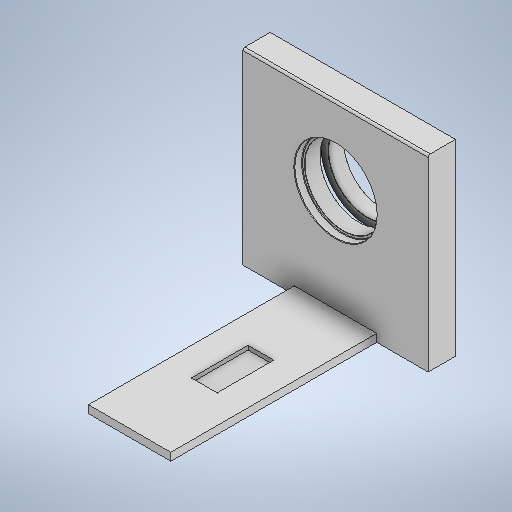
# Autodesk Inventor part: Gantry mssd
Saved by Autodesk Inventor 2025.2 (Build 292293000, 293)
## iProperties
Created: 2025-04-03
Part Number: Gantry mssd
Material: Generic
Document SubType Name: Modeling
Designer: NIKHIL
Density: 1 g/cm^3
Appearance: Default
Author: NIKHIL
Autodesk Inventor part; units mm, degrees
sketch "Sketch1" plane through (0, 0, 0) normal (0, 0, 1) x (1, 0, 0)
  circle A0 centre (0, 0) radius 375
  circle A1 centre (0, 0) radius 450
  dimension "d0" = 750
  dimension "d2" = 900
  constraints: 2 centre point, 2 coincident
  measures "d0" diameter of A0
  measures "d2" diameter of A1
extrude "Extrusion1" add sketch "Sketch1" along normal blind 150
ref_plane "Work Plane1" through (0, 0, -80) normal (0, 0, -1) x (-1, 0, 0)
sketch "Sketch2" plane through (0, 0, -80) normal (0, 0, -1) x (-1, 0, 0)
  circle A0 centre (0, 0) radius 375
  circle A1 centre (0, 0) radius 450
  constraints: 2 centre point, 2 coincident
extrude "Extrusion2" add sketch "Sketch2" along normal blind 150
ref_plane "Work Plane2" through (0, 400, 0) normal (0, 1, 0) x (-1, 0, 0)
sketch "Sketch5" plane through (0, 0, 0) normal (1, 0, 0) x (0, 1, 0)
  line L0 (450, 0) -> (450, 150) projected
  line L1 (450, 70) -> (465, 70)
  line L2 (465, 70) -> (465, 80)
  line L3 (465, 80) -> (450, 80)
  line L4 (450, 80) -> (450, 70)
  line L5 (0, -306) -> (0, 226) projected
  line L6 (450, -80) -> (450, -230) projected
  line L7 (450, -150) -> (465, -150)
  line L8 (465, -150) -> (465, -160)
  line L9 (465, -160) -> (450, -160)
  line L10 (450, -160) -> (450, -150)
  point P0 (0, 0)
  dimension "d11" = 15
  dimension "d12" = 10
  dimension "d14" = 15
  dimension "d15" = 10
  constraints: 16 end point, 4 parallel, 2 horizontal, 2 perpendicular, 2 point on line
  measures "d11" distance of L3.end L2.end
  measures "d12" distance of L2.end L1.end
  measures "d14" distance of L8.end L9.end
  measures "d15" distance of L7.end L8.end
revolve "Revolution1" add sketch "Sketch5" angle 360 about axis through (0, 0, -10) along (0, 0, 1)
ref_plane "Work Plane3" through (0, 0, -40) normal (0, 0, 1) x (1, 0, 0)
ref_plane "Work Plane4" through (0, 0, 150) normal (0, 0, 1) x (1, 0, 0)
sketch "Sketch11" plane through (0, 0, 150) normal (0, 0, 1) x (1, 0, 0)
  circle A0 centre (0, 0) radius 400
  line L0 (-900, 750) -> (900, 750)
  line L1 (900, 750) -> (900, -750)
  line L2 (900, -750) -> (-900, -750)
  line L3 (-900, -750) -> (-900, 750)
  line L4 (-900, 750) -> (900, -750) construction
  line L5 (900, 750) -> (-900, -750) construction
  dimension "d33" = 800
  dimension "d34" = 1800
  dimension "d35" = 1500
  constraints: 12 end point, 2 midpoint, 2 parallel, 1 centre point, 1 coincident, 1 horizontal, 1 perpendicular
  measures "d33" diameter of A0
  measures "d34" distance of L1.end L2.end
  measures "d35" distance of L0.end L1.end
extrude "Extrusion5" add sketch "Sketch11" along normal blind 75
fillet "Fillet1" radius 5 1 edges at (-400, 0, 225)
fillet "Fillet2" radius 5 1 edges at (-400, 0, 150)
fillet "Fillet3" radius 2 1 edges at (-375, 0, 150)
fillet "Fillet4" radius 2 1 edges at (-375, 0, 0)
fillet "Fillet5" radius 2 1 edges at (375, 0, -80)
fillet "Fillet6" radius 2 1 edges at (375, 0, -230)
fillet "Fillet7" radius 2 1 edges at (-450, 0, 0)
fillet "Fillet8" radius 2 2 edges at (450, 0, -80) (450, 0, -230)
fillet "Fillet9" radius 20 1 edges at (0, 750, 225)
sketch "Sketch15" plane through (-900, -750, 150) normal (0, -1, 0) x (1, 0, 0)
  line L0 (1800, 75) -> (1800, 55) projected
  line L1 (0, 0) -> (1800, 0) projected
  line L2 (1800, 75) -> (0, 75)
  line L3 (0, 75) -> (0, 0)
  line L4 (0, 0) -> (1800, 0)
  line L5 (1800, 0) -> (1800, 75)
  point P0 (900, -150)
  constraints: 8 end point, 2 parallel, 1 horizontal, 1 perpendicular
extrude "Extrusion7" add sketch "Sketch15" along normal blind 325
sketch "Sketch16" plane through (0, 0, 225) normal (0, 0, 1) x (1, 0, 0)
  line L0 (-900, -1075) -> (900, -1075) projected
  line L1 (0, -1075) -> (400, -1075)
  line L2 (400, -1075) -> (400, -1000)
  line L3 (400, -1000) -> (-400, -1000)
  line L4 (-400, -1000) -> (-400, -1075)
  line L5 (-400, -1075) -> (0, -1075)
  point P0 (0, 0)
  dimension "d64" = 400
  dimension "d65" = 75
  dimension "d66" = 800
  constraints: 10 end point, 3 perpendicular, 2 point on line, 1 collinear, 1 midpoint
  measures "d64" distance of L1.start L1.end
  measures "d65" distance of L1.end L2.end
  measures "d66" distance of L2.end L3.end
extrude "Extrusion8" add sketch "Sketch16" along normal blind 2000
sketch "Sketch17" plane through (-400, -1000, 225) normal (0, 1, 0) x (1, 0, 0)
  line L0 (400, -725) -> (525, -725)
  line L1 (525, -725) -> (525, -1275)
  line L2 (525, -1275) -> (275, -1275)
  line L3 (275, -1275) -> (275, -725)
  line L4 (275, -725) -> (400, -725)
  line L5 (-500, 0) -> (1300, 0) projected
  point P0 (400, 225)
  point P1 (-480, 0)
  point P2 (1280, 0)
  dimension "d72" = 725
  constraints: 10 end point, 4 perpendicular, 1 horizontal, 1 point on line
  measures "d72" distance between parallel lines of L4 L5
extrude "Extrusion9" cut sketch "Sketch17" against normal blind 40
sketch "Sketch18" plane through (0, 0, 150) normal (0, 0, -1) x (-1, 0, 0)
  line L0 (900, -1075) -> (880, -1075) projected
  line L1 (-900, 750) -> (900, 750)
  line L2 (900, 750) -> (900, -1075)
  line L3 (900, -1075) -> (-900, -1075)
  line L4 (-900, -1075) -> (-900, 750)
  line L5 (-875, 725) -> (875, 725)
  line L6 (875, 725) -> (875, -1050)
  line L7 (875, -1050) -> (-875, -1050)
  line L8 (-875, -1050) -> (-875, 725)
  line L9 (-850, 700) -> (850, 700)
  line L10 (850, 700) -> (850, -1025)
  line L11 (850, -1025) -> (-850, -1025)
  line L12 (-850, -1025) -> (-850, 700)
  line L13 (-825, 675) -> (825, 675)
  line L14 (825, 675) -> (825, -1000)
  line L15 (825, -1000) -> (-825, -1000)
  line L16 (-825, -1000) -> (-825, 675)
  point P0 (0, 0)
  constraints: 32 end point, 8 parallel, 4 horizontal, 4 perpendicular
extrude "Extrusion10" add sketch "Sketch18" along normal blind 190
sketch "Sketch20" plane through (0, 0, 150) normal (0, 0, -1) x (-1, 0, 0)
  line L0 (0, -675) -> (825, -675)
  line L1 (825, -675) -> (825, -700)
  line L2 (825, -700) -> (0, -700)
  line L3 (0, -503.4054) -> (0, -575.6964) construction
  line L4 (0, -775) -> (825, -775)
  line L5 (825, -775) -> (825, -800)
  line L6 (825, -800) -> (0, -800)
  line L7 (0, -875) -> (825, -875)
  line L8 (825, -875) -> (825, -900)
  line L9 (825, -900) -> (0, -900)
  line L10 (0, -675) -> (-825, -675)
  line L11 (-825, -675) -> (-825, -700)
  line L12 (-825, -700) -> (0, -700)
  line L13 (0, -775) -> (-825, -775)
  line L14 (-825, -775) -> (-825, -800)
  line L15 (-825, -800) -> (0, -800)
  line L16 (0, -875) -> (-825, -875)
  line L17 (-825, -875) -> (-825, -900)
  line L18 (-825, -900) -> (0, -900)
  line L19 (720, -675) -> (720, 675)
  line L20 (695, 675) -> (695, -675)
  line L21 (720, 675) -> (695, 675)
  line L22 (825, 675) -> (-825, 675) construction
  line L23 (-720, -675) -> (-720, 675)
  line L24 (-695, 675) -> (-695, -675)
  line L25 (-720, 675) -> (-695, 675)
  point P0 (0, 0)
  dimension "d86" = 100
  constraints: 50 end point, 10 symmetric about line, 3 vertical, 2 perpendicular, 2 point on line, 1 collinear, 1 horizontal, 1 parallel, 14 other
  measures "d86" distance of L0.start L4.start
extrude "Extrusion11" add sketch "Sketch20" along normal blind 190
body "Solid1"
